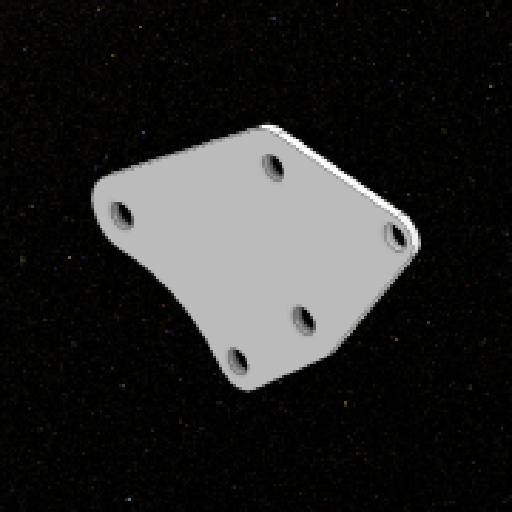
# Autodesk Inventor part: odom_pod
Saved by Autodesk Inventor 2024 (Build 280153000, 153)
## iProperties
Created: 2024-02-24
Part Number: odom_pod
Material: Acetal Resin, White
Document SubType Name: Modeling
Designer: Averey Ku
Density: 1.425 g/cm^3
Appearance: Smooth - White
Author: Averey Ku
Autodesk Inventor part; units mm, degrees
ref_plane "YZ Plane" through (0, 0, 0) normal (1, 0, 0) x (0, 1, 0)
ref_plane "XZ Plane" through (0, 0, 0) normal (0, 1, 0) x (-1, 0, 0)
ref_plane "XY Plane" through (0, 0, 0) normal (0, 0, 1) x (1, 0, 0)
sketch "Sketch1" plane through (0, 0, 0) normal (0, 0, 1) x (1, 0, 0)
  circle A0 centre (0, 0) radius 2.2479
  circle A1 centre (38.1, 0) radius 2.2479
  circle A2 centre (31.7852, 24.6214) radius 2.0955
  arc A3 (-3.8886, 5.0201) -> (-0.1468, -6.3483) centre (0, 0) ccw
  arc A4 (34.9548, 30.1237) -> (27.8966, 29.6414) centre (31.7852, 24.6214) ccw
  line L0 (-3.8886, 5.0201) -> (27.8966, 29.6414)
  line L1 (38.1, 0) -> (63.5, 0) construction
  circle A5 centre (22.225, -19.05) radius 2.0955
  arc A6 (17.6269, -20.2907) -> (25.681, -22.3268) centre (22.225, -19.05) ccw
  arc A7 (17.6269, -20.2907) -> (-0.1468, -6.3483) centre (-0.5827, -25.2041) ccw
  line L2 (37.8478, -9.4949) -> (25.681, -22.3268)
  circle A8 centre (60.325, 11.1125) radius 2.2479
  arc A9 (62.3683, 7.8968) -> (62.2268, 14.4139) centre (60.325, 11.1125) ccw
  line L3 (62.2268, 14.4139) -> (34.9548, 30.1237)
  line L4 (62.3683, 7.8968) -> (47.4674, -1.5713)
  arc A10 (47.4674, -1.5713) -> (37.8478, -9.4949) centre (74.7114, -44.448) ccw
  point P0 (42.1679, -4.9387)
  dimension "d0" = 4.4958
  dimension "d5" = 12.7
  dimension "d6" = 12.7
  dimension "d14" = 9.525
  dimension "d16" = 7.62
  dimension "d17" = 50.8
  constraints: 12 point on circle, 11 centre point, 10 end point, 10 tangent, 6 coincident, 2 point on line, 1 horizontal, 1 other
  measures "d0" diameter of A0
  measures "d5" diameter of A3
  measures "d6" diameter of A4
  measures "d14" diameter of A6
  measures "d16" diameter of A9
  measures "d17" radius of A10
extrude "Extrusion1" add sketch "Sketch1" along normal blind 1.5875
body "Solid1"
